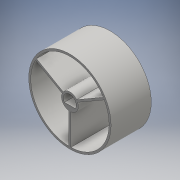
# Autodesk Inventor part: Wheel_Actual-wheel-ENES100OSVproject-spencermical-3-3-16_thursday-1-17am-freshmanyear-springsemester
Saved by Autodesk Inventor 2016 (Build 200138000, 138)
## iProperties
Created: 2016-03-03
Part Number: Wheel_Actual-wheel-ENES100OSVproject-spencermical-3-3-16_thursday-1-17am-freshmanyear-springsemester
Material: Generic
Document SubType Name: Modeling
Designer: Spencer
Density: 1 g/cm^3
Appearance: Default
Author: Spencer
Autodesk Inventor part; units mm, degrees
ref_plane "YZ Plane" through (0, 0, 0) normal (1, 0, 0) x (0, 1, 0)
ref_plane "XZ Plane" through (0, 0, 0) normal (0, 1, 0) x (-1, 0, 0)
ref_plane "XY Plane" through (0, 0, 0) normal (0, 0, 1) x (1, 0, 0)
sketch "Sketch1" plane through (0, 0, 0) normal (0, 1, 0) x (-1, 0, 0)
  circle A0 centre (0, 0) radius 61.5
  dimension "d0" = 123
  constraints: 1 centre point, 1 coincident
  measures "d0" diameter of A0
extrude "Extrusion1" add sketch "Sketch1" along normal blind 60
thread "Thread1" size "M125x8" class "6g" standard "ANSI Metric M Profile" full length
sketch "Sketch2" plane through (0, 60, 0) normal (0, 1, 0) x (1, 0, 0)
  arc A0 (-8.1881, 5) -> (8.1881, 5) centre (0, 0) ccw
  line L0 (-8.1881, 5) -> (8.1881, 5)
  dimension "d5" = 19.188
  dimension "d6" = 5
  constraints: 2 end point, 2 point on circle, 1 centre point, 1 coincident, 1 horizontal
  measures "d5" diameter of A0
  measures "d6" distance from line of point (0, 0) L0
extrude "Extrusion2" cut sketch "Sketch2" against normal up to surface (60 mm away)
sketch "Sketch3" plane through (0, 60, 0) normal (0, 1, 0) x (1, 0, 0)
  line L0 (-8.1881, 5) -> (8.1881, 5) projected
  arc A0 (-8.1881, 5) -> (8.1881, 5) centre (0, 0) ccw projected
  circle A1 centre (0, 0) radius 61.5 projected
  line L1 (-1.5, 58.4808) -> (-1.5, 12.5044)
  line L2 (1.5, 58.4808) -> (1.5, 12.5044)
  line L3 (-49.8958, -30.5394) -> (-10.0791, -7.5512)
  line L4 (-51.3958, -27.9413) -> (-11.5791, -4.9531)
  line L5 (51.3958, -27.9413) -> (11.5791, -4.9531)
  line L6 (49.8958, -30.5394) -> (10.0791, -7.5512)
  arc A2 (11.5791, -4.9531) -> (1.5, 12.5044) centre (0, 0) ccw
  arc A3 (-1.5, 12.5044) -> (-11.5791, -4.9531) centre (0, 0) ccw
  arc A4 (-10.0791, -7.5512) -> (10.0791, -7.5512) centre (0, 0) ccw
  arc A5 (-49.8958, -30.5394) -> (49.8958, -30.5394) centre (0, 0) ccw
  arc A6 (51.3958, -27.9413) -> (1.5, 58.4808) centre (0, 0) ccw
  arc A7 (-1.5, 58.4808) -> (-51.3958, -27.9413) centre (0, 0) ccw
  dimension "d11" = 3
  dimension "d14" = 360
  constraints: 12 end point, 12 point on circle, 6 centre point, 2 vertical, 1 coincident, 1 parallel, 19 other
  measures "d11" distance between parallel lines of L2 L1
extrude "Extrusion3" cut sketch "Sketch3" against normal through all contours L1 A3 L4 A7 | A6 L5 A2 L2 | L3 A4 L6 A5
body "Solid1"
